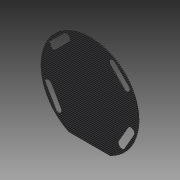
# Autodesk Inventor part: Bottom Plate
Saved by Autodesk Inventor 2015 (Build 190159000, 159)
## iProperties
Created: 2016-08-08
Part Number: Bottom Plate
Material: Generic
Document SubType Name: Modeling
Designer: James Yelland
Density: 1 g/cm^3
Appearance: Default
Author: James Yelland
Autodesk Inventor part; units mm, degrees
ref_plane "YZ Plane" through (0, 0, 0) normal (1, 0, 0) x (0, 1, 0)
ref_plane "XZ Plane" through (0, 0, 0) normal (0, 1, 0) x (-1, 0, 0)
ref_plane "XY Plane" through (0, 0, 0) normal (0, 0, 1) x (1, 0, 0)
sketch "Sketch1" plane through (0, 0, 0) normal (0, 1, 0) x (-1, 0, 0)
  line L0 (-84.8705, -49) -> (-74.3705, -67.1865)
  line L1 (-64.8083, -69.7487) -> (-63.9423, -69.2487)
  line L2 (-61.3801, -59.6865) -> (-82.3801, -23.3135)
  line L3 (-91.9423, -20.7513) -> (-92.8083, -21.2513)
  line L4 (-95.3705, -30.8135) -> (-84.8705, -49)
  arc A0 (-63.9423, -69.2487) -> (-61.3801, -59.6865) centre (-67.4423, -63.1865) ccw
  arc A1 (-74.3705, -67.1865) -> (-64.8083, -69.7487) centre (-68.3083, -63.6865) ccw
  arc A2 (-92.8083, -21.2513) -> (-95.3705, -30.8135) centre (-89.3083, -27.3135) ccw
  arc A3 (-82.3801, -23.3135) -> (-91.9423, -20.7513) centre (-88.4423, -26.8135) ccw
  line L5 (84.8705, -49) -> (95.3705, -30.8135)
  line L6 (92.8083, -21.2513) -> (91.9423, -20.7513)
  line L7 (82.3801, -23.3135) -> (61.3801, -59.6865)
  line L8 (63.9423, -69.2487) -> (64.8083, -69.7487)
  line L9 (74.3705, -67.1865) -> (84.8705, -49)
  arc A4 (91.9423, -20.7513) -> (82.3801, -23.3135) centre (88.4423, -26.8135) ccw
  arc A5 (95.3705, -30.8135) -> (92.8083, -21.2513) centre (89.3083, -27.3135) ccw
  arc A6 (64.8083, -69.7487) -> (74.3705, -67.1865) centre (68.3083, -63.6865) ccw
  arc A7 (61.3801, -59.6865) -> (63.9423, -69.2487) centre (67.4423, -63.1865) ccw
  line L10 (69.2965, 69.2965) -> (54.4472, 84.1457)
  line L11 (44.5477, 84.1457) -> (43.8406, 83.4386)
  line L12 (43.8406, 73.5391) -> (73.5391, 43.8406)
  line L13 (83.4386, 43.8406) -> (84.1457, 44.5477)
  line L14 (84.1457, 54.4472) -> (69.2965, 69.2965)
  arc A8 (43.8406, 83.4386) -> (43.8406, 73.5391) centre (48.7904, 78.4889) ccw
  arc A9 (54.4472, 84.1457) -> (44.5477, 84.1457) centre (49.4975, 79.196) ccw
  arc A10 (84.1457, 44.5477) -> (84.1457, 54.4472) centre (79.196, 49.4975) ccw
  arc A11 (73.5391, 43.8406) -> (83.4386, 43.8406) centre (78.4889, 48.7904) ccw
  line L15 (-69.2965, 69.2965) -> (-84.1457, 54.4472)
  line L16 (-84.1457, 44.5477) -> (-83.4386, 43.8406)
  line L17 (-73.5391, 43.8406) -> (-43.8406, 73.5391)
  line L18 (-43.8406, 83.4386) -> (-44.5477, 84.1457)
  line L19 (-54.4472, 84.1457) -> (-69.2965, 69.2965)
  arc A12 (-83.4386, 43.8406) -> (-73.5391, 43.8406) centre (-78.4889, 48.7904) ccw
  arc A13 (-84.1457, 54.4472) -> (-84.1457, 44.5477) centre (-79.196, 49.4975) ccw
  arc A14 (-44.5477, 84.1457) -> (-54.4472, 84.1457) centre (-49.4975, 79.196) ccw
  arc A15 (-43.8406, 73.5391) -> (-43.8406, 83.4386) centre (-48.7904, 78.4889) ccw
  line L20 (0, 0) -> (44.3749, -95.1623)
  line L21 (0, 0) -> (-44.3749, -95.1623)
  line L22 (-44.3749, -95.1623) -> (44.3749, -95.1623)
  arc A16 (44.3749, -95.1623) -> (-44.3749, -95.1623) centre (0, 0) ccw
  line L23 (0, 0) -> (-58.6899, 58.6899)
  line L24 (0, 0) -> (58.6899, 58.6899)
  line L25 (0, 0) -> (71.8801, -41.5)
  line L26 (0, 0) -> (-71.8801, -41.5)
  point P0 (-38.8909, -78.4889)
  point P1 (-85.8801, -17.2513)
  point P2 (-89.0955, -49.4975)
  point P3 (98.8705, -24.7513)
  point P4 (85.8801, -17.2513)
  point P5 (38.8909, -78.4889)
  point P6 (49.4975, -89.0955)
  point P7 (49.4975, 89.0955)
  point P8 (38.8909, 78.4889)
  point P9 (78.4889, 38.8909)
  point P10 (89.0955, 49.4975)
  point P11 (-89.0955, 49.4975)
  point P12 (-78.4889, 38.8909)
  point P13 (-38.8909, 78.4889)
  point P14 (-49.4975, 89.0955)
  constraints: 54 end point, 34 point on circle, 24 point on line, 17 centre point, 4 midpoint, 1 coincident
extrude "Extrusion1" add sketch "Sketch1" along normal blind 2
body "Solid1"
